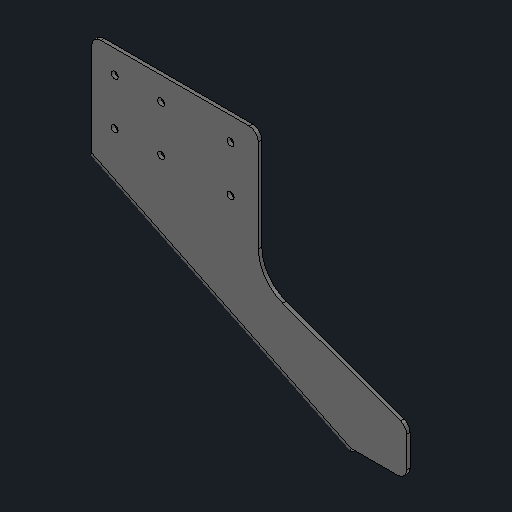
# Autodesk Inventor part: Model-2_Sheet-LH
Saved by Autodesk Inventor 2025.1 (Build 291241000, 241)
## iProperties
RuleStatus: InUse
Created: 2026-02-13
Part Number: Model-2_Sheet-LH
User Status: Released
Material: SS304
Document SubType Name: Sheet Metal
Designer: Desktop -24
Density: 7.99949 g/cm^3
Sheet Metal Rule: 3/8" (3.150 Die)
Appearance: Semi-Polished(1)
AfterDocNew0: Mat. Selection
encoded128: ÌSheet Metal (in)XÎ
Family: SS304
Author: Desktop -24
Revision Number: 0
Autodesk Inventor part; units mm, degrees
ref_plane "YZ Plane" through (0, 0, 0) normal (1, 0, 0) x (0, 1, 0)
ref_plane "XZ Plane" through (0, 0, 0) normal (0, 1, 0) x (-1, 0, 0)
ref_plane "XY Plane" through (0, 0, 0) normal (0, 0, 1) x (1, 0, 0)
sketch "Sketch1" plane through (0, 0, 0) normal (0, 0, 1) x (1, 0, 0)
  line L0 (-203.2, 0) -> (203.2, 0)
  line L1 (-228.6, -279.4) -> (-228.6, -25.4)
  line L2 (228.6, -25.4) -> (228.6, -279.4)
  line L3 (295.4508, -374.8728) -> (618.2873, -492.3757)
  line L4 (635, -516.2439) -> (635, -600.0586)
  line L5 (609.6, -625.4586) -> (482.6, -625.4586)
  line L6 (482.6, -625.4586) -> (-228.6, -279.4)
  arc A0 (228.6, -279.4) -> (295.4508, -374.8728) centre (330.2, -279.4) ccw
  line L7 (-165.1, -190.5) -> (-38.1, -190.5) construction
  line L8 (-38.1, -190.5) -> (-38.1, -63.5) construction
  line L9 (-38.1, -63.5) -> (-165.1, -63.5) construction
  line L10 (-165.1, -63.5) -> (-165.1, -190.5) construction
  line L11 (-165.1, -190.5) -> (-38.1, -63.5) construction
  line L12 (-38.1, -190.5) -> (-165.1, -63.5) construction
  circle A1 centre (-165.1, -63.5) radius 9.525
  circle A2 centre (-38.1, -63.5) radius 9.525
  circle A3 centre (-38.1, -190.5) radius 9.525
  circle A4 centre (-165.1, -190.5) radius 9.525
  circle A5 centre (152.4, -63.5) radius 9.6564
  circle A6 centre (152.4, -190.5) radius 9.525
  arc A7 (635, -516.2439) -> (618.2873, -492.3757) centre (609.6, -516.2439) ccw
  arc A8 (609.6, -625.4586) -> (635, -600.0586) centre (609.6, -600.0586) ccw
  arc A9 (228.6, -25.4) -> (203.2, 0) centre (203.2, -25.4) ccw
  arc A10 (-203.2, 0) -> (-228.6, -25.4) centre (-203.2, -25.4) ccw
  point P0 (0, 0)
  point P1 (-228.6, 0)
  point P2 (228.6, 0)
  point P3 (0, 0)
  point P4 (635, -498.4586)
  point P5 (635, -625.4586)
  point P6 (-101.6, -127)
  point P7 (635, -558.1512)
  point P8 (546.1, -625.4586)
  dimension "d0" = 127
  dimension "d1" = 457.2
  dimension "d2" = 101.6
  dimension "d3" = 110
  dimension "d5" = 152.4
  dimension "d7" = 19.05
  dimension "d8" = 127
  dimension "d9" = 127
  dimension "d10" = 63.5
  dimension "d11" = 63.5
  dimension "d12" = 76.2
  dimension "d13" = 635
  dimension "d14" = 25.4
  dimension "d16" = 254
  measures "d0" distance of point (635, -498.459) point (635, -625.459)
  measures "d1" distance of point (-228.6, 0) point (228.6, 0)
  measures "d2" radius of A0
  measures "d3" angle of L3 L2
  measures "d5" distance of point (635, -625.459) L5.end
  measures "d7" diameter of A2
  measures "d8" distance of L8.end L9.end
  measures "d9" distance of L9.end L7.start
  measures "d10" distance between parallel lines of L0 L9
  measures "d11" distance between parallel lines of L1 L10
  measures "d12" distance from line of A5.centre L2
  measures "d13" horizontal distance of point (635, -558.151) point (0, 0)
  measures "d14" radius of A7
  measures "d16" distance of L1.start L1.end
extrude "Plate1" add sketch "Sketch1" along normal blind 9.525
sketch "Sketch2" plane through (-234.379, -291.2766, -13.208) normal (-0.4375367, -0.8992006, 0) x (0.8992006, -0.4375367, 0)
  line L0 (790.9248, 0) -> (0, 0)
  line L1 (0, 0) -> (0, -24.892)
  line L2 (0, -24.892) -> (790.9248, -24.892)
  line L3 (790.9248, -24.892) -> (790.9248, 0)
  constraints: 6 end point, 1 horizontal, 1 perpendicular, 1 vertical
edge flange "Flange1" height 38.1 angle 90 thickness 9.525 bend radius 13.208 thickness toward (-0.4375367, -0.8992006, 0) relief tear relief width 9.525 relief depth 4.7625 edges at (127, -452.4293, 0) wall of the first edge with corners at (476.821, -637.3352, -13.208) (-234.379, -291.2766, -13.208) (-234.379, -291.2766, -38.1) (476.821, -637.3352, -38.1)
bend "Bend1"
corner "Corner1"
equation "\"d15\" = Thickness"
equation "\"d19\" = BendReliefWidth"
equation "\"d20\" = BendReliefDepth"
equation "\"d21\" = MinimumRemnant"
equation "\"d22\" = TransitionRadius"
equation "\"d25\" = BendRadius"
equation "\"d26\" = CornerReliefSize"
equation "\"d27\" = GapSize"
equation "\"d28\" = JacobiRadiusSize"
equation "\"BendReliefWidth\" = Thickness"
equation "\"BendReliefDepth\" = 0.5 * Thickness"
equation "\"CornerReliefSize\" = 4 * Thickness"
equation "\"MinimumRemnant\" = 2 * Thickness"
equation "\"TransitionRadius\" = BendRadius"
equation "\"JacobiRadiusSize\" = Thickness"
equation "\"GapSize\" = Thickness"
equation "\"Thickness\" = 9.525"
equation "\"BendRadius\" = 13.208"
body "Solid1"
